Autodesk Fusion 360 part; units mm, degrees
(part 2 of 2)
component "Big_relay" placed x (0, -1, 0) y (1, 0, 0) z (0, 0, 1) at (-21.5, 191.5, 55)
component "Switch_holder" placed x (0, -1, 0) y (1, 0, 0) z (0, 0, 1) at (52.5, 40, 108)
equation "d65 = 60 mm - ( 10.1 * 2 ) * 1 mm"
equation "d73 = 60 mm - ( 10 * 2 ) * 1 mm"
named bodies: "Breadbord", "Arduino", "Mosfet", "Big_relay", "Mosfet (1)", "Mosfet (2)", "lcd"
